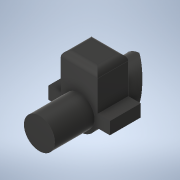
# Autodesk Inventor part: スライド
Saved by Autodesk Inventor 2020 (Build 240168000, 168)
## iProperties
Created: 2020-02-12
Part Number: スライド
Material: 一般
Document SubType Name: Modeling
Designer: 久保寺 真仁
Density: 1 g/cm^3
Appearance: 既定
Author: 久保寺 真仁
Autodesk Inventor part; units mm, degrees
sketch "スケッチ1" plane through (0, 0, 0) normal (0, 0, 1) x (1, 0, 0)
  point P0 (0, 0)
sketch "スケッチ2" plane through (0, 0, 0) normal (0, 0, 1) x (1, 0, 0)
  circle A0 centre (0, 0) radius 2.5
  dimension "d0" = 5
  constraints: 1 centre point, 1 coincident
  measures "d0" diameter of A0
extrude "押し出し1" add sketch "スケッチ2" along normal blind 6.5
sketch "スケッチ3" plane through (0, 0, 0) normal (0, 0, -1) x (-1, 0, 0)
  circle A0 centre (0, 0) radius 3
  dimension "d3" = 6
  constraints: 1 centre point, 1 coincident
  measures "d3" diameter of A0
extrude "押し出し2" add sketch "スケッチ3" along normal blind 10
sketch "スケッチ4" plane through (0, 0, 0) normal (0, 0, 1) x (1, 0, 0)
  circle A0 centre (0, 0) radius 3 projected
  point P0 (0, 3)
  constraints: 1 coincident, 1 vertical alignment, 1 other
ref_plane "作業平面2" through (0, 0, 0) normal (0, 1, 0) x (-1, 0, 0)
ref_plane "作業平面1" through (0, 3, 0) normal (0, 1, 0) x (-1, 0, 0)
sketch "スケッチ5" plane through (0, 0, 0) normal (0, 1, 0) x (-1, 0, 0)
  line L0 (5, -5) -> (-5, -5)
  line L1 (-5, -5) -> (-5, 0)
  line L2 (-5, 0) -> (5, 0)
  line L3 (5, 0) -> (5, -5)
  point P0 (0, 0)
  dimension "d7" = 10
  dimension "d8" = 5
  dimension "d9" = 5
  constraints: 8 end point, 2 parallel, 1 horizontal, 1 perpendicular
  measures "d7" distance between parallel lines of L1 L3
  measures "d8" distance between parallel lines of L0 L2
  measures "d9" distance from line of L1 point (0, 0)
extrude "押し出し3" add sketch "スケッチ5" along normal mid plane 2
sketch "スケッチ6" plane through (0, 0, 0) normal (0, 1, 0) x (-1, 0, 0)
  line L0 (5, -5) -> (2.8284, -5) projected
  line L1 (-2.8284, 0) -> (-5, 0) projected
  line L2 (3, -5) -> (-3.9142, -5)
  line L3 (-3.9142, -5) -> (-3.9142, 0)
  line L4 (-3.9142, 0) -> (3, 0)
  line L5 (3, 0) -> (3, -5)
  line L6 (3.5037, -5) -> (-3, -5)
  line L7 (-3, -5) -> (-3, 0)
  line L8 (-3, 0) -> (3.5037, 0)
  line L9 (3.5037, 0) -> (3.5037, -5)
  point P0 (0, 0)
  dimension "d12" = 6
  dimension "d13" = 3
  constraints: 16 end point, 4 parallel, 3 point on line, 2 horizontal, 2 perpendicular, 1 midpoint
  measures "d12" distance between parallel lines of L7 L5
  measures "d13" distance from line of L7 point (0, 0)
extrude "押し出し4" add sketch "スケッチ6" along normal blind 7 contours L0 L2 L7 L1 L4 L5
fillet "フィレット1" radius 1 4 edges at (0, 7, 0) (-3, 7, -2.5) (0, 7, -5) (3, 7, -2.5)
sketch "スケッチ7" plane through (0, 0, -10) normal (0, 0, -1) x (-1, 0, 0)
  arc A0 (2.8284, -1) -> (-2.8284, -1) centre (0, 0) ccw projected
  point P0 (3, 0)
  constraints: 1 point on circle
ref_plane "作業平面3" through (-3, 0, -10) normal (-1, 0, 0) x (0, -1, 0)
sketch "スケッチ12" plane through (0, 0, -10) normal (0, 0, -1) x (-1, 0, 0)
  circle A0 centre (0, 0) radius 3 construction
  arc A1 (2.8284, -1) -> (-2.8284, -1) centre (0, 0) ccw construction
  line L0 (-0.7765, 2.8978) -> (0.7765, -2.8978) construction
  circle A2 centre (0, 0) radius 3 construction
  line L1 (3, 0) -> (-3, 0) construction
  dimension "d22" = 105
  constraints: 5 point on circle, 4 end point, 2 coincident, 1 centre point, 1 midpoint, 1 other
  measures "d22" angle of L0 L1
ref_plane "作業平面6" through (0.7765, 2.8978, -10) normal (-0.2588, -0.9659, 0) x (0.9659, -0.2588, 0)
sketch "スケッチ13" plane through (0.7765, 2.8978, -10) normal (-0.2588, -0.9659, 0) x (0.9659, -0.2588, 0)
  line L0 (-3, 0) -> (3, 0) projected
  line L1 (3, 0) -> (3, 3)
  line L2 (3, 5) -> (3, 0) projected
  line L3 (3, 0) -> (-1, 0)
  line L4 (-1, 0) -> (3, 3)
  point P0 (0, 10)
  dimension "d23" = 3
  dimension "d24" = 4
  constraints: 6 end point, 2 point on line
  measures "d23" distance of L0.end L1.end
  measures "d24" distance of L2.end L3.end
extrude "押し出し6" cut sketch "スケッチ13" along normal through all
equation "\"d9\" = 0.5 * d7"
equation "\"d13\" = 0.5 * d12"
